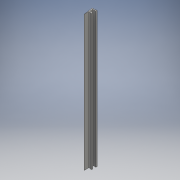
# Autodesk Inventor part: LedStripHolder
Saved by Autodesk Inventor 2016 (Build 200138000, 138)
## iProperties
Created: 2015-05-25
Part Number: LedStripHolder
Material: Generic
Document SubType Name: Modeling
Designer: Jack
Density: 1 g/cm^3
Appearance: Default
Author: Jack
Autodesk Inventor part; units mm, degrees
ref_plane "YZ Plane" through (0, 0, 0) normal (1, 0, 0) x (0, 1, 0)
ref_plane "XZ Plane" through (0, 0, 0) normal (0, 1, 0) x (-1, 0, 0)
ref_plane "XY Plane" through (0, 0, 0) normal (0, 0, 1) x (1, 0, 0)
sketch "Sketch1" plane through (0, 0, 0) normal (0, 0, 1) x (1, 0, 0)
  line L0 (0, 0) -> (-1.6865, 12)
  line L1 (-1.6865, 12) -> (0, 12)
  line L2 (0, 12) -> (0, 0)
  dimension "d0" = 8
  dimension "d1" = 12
  constraints: 6 end point, 1 horizontal, 1 perpendicular
  measures "d0" angle of L2 L0
  measures "d1" distance of L1.end L0.start
extrude "Extrusion1" add sketch "Sketch1" along normal blind 175
sketch "Sketch2" plane through (0, 0, 175) normal (0, 0, 1) x (1, 0, 0)
  line L0 (0, 0) -> (0, 12) projected
  line L1 (0, 12) -> (-1.6865, 12) projected
  line L2 (0, 12) -> (2, 12)
  line L3 (2, 12) -> (2.5, 12.5)
  line L4 (2.5, 12.5) -> (4, 12.5)
  line L5 (4, 12.5) -> (4, 11)
  line L6 (4, 11) -> (0, 11)
  line L7 (0, 7) -> (4, 7)
  line L8 (4, 7) -> (4, 5.5)
  line L9 (4, 5.5) -> (2.5, 5.5)
  line L10 (2.5, 5.5) -> (2, 6)
  line L11 (2, 6) -> (0, 6)
  dimension "d4" = 2
  dimension "d5" = 4
  dimension "d6" = 135
  dimension "d7" = 0.5
  dimension "d8" = 1.5
  dimension "d9" = 135
  dimension "d10" = 4
  dimension "d11" = 1
  constraints: 20 end point, 5 perpendicular, 4 equal length, 3 horizontal, 3 point on line, 1 midpoint
  measures "d4" distance of L2.start L2.end
  measures "d5" distance of L5.end L6.end
  measures "d6" angle of L3 L2
  measures "d7" horizontal distance of L3.end L2.end
  measures "d8" distance of L4.end L5.end
  measures "d9" angle of L11 L10
  measures "d10" distance between parallel lines of L6 L7
  measures "d11" distance between parallel lines of L1 L6
extrude "Extrusion2" add sketch "Sketch2" against normal up to surface (175 mm away)
body "Solid1"
